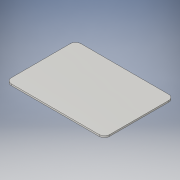
# Autodesk Inventor part: Panel
Saved by Autodesk Inventor 2016 (Build 200138000, 138)
## iProperties
Created: 2016-03-01
Part Number: Panel
Material: Acetal Resin, White
Document SubType Name: Modeling
Designer: agmle
Mass: 839 g
Surface Area: 2036.95 cm^2
Volume: 588.772 cm^3
Density: 1.425 g/cm^3
Appearance: Smooth - White
Author: agmle
Autodesk Inventor part; units mm, degrees
ref_plane "YZ Plane" through (0, 0, 0) normal (1, 0, 0) x (0, 1, 0)
ref_plane "XZ Plane" through (0, 0, 0) normal (0, 1, 0) x (-1, 0, 0)
ref_plane "XY Plane" through (0, 0, 0) normal (0, 0, 1) x (1, 0, 0)
sketch "Sketch1" plane through (0, 0, 0) normal (0, 1, 0) x (-1, 0, 0)
  line L0 (166.5, -132) -> (-166.5, -132)
  line L1 (-186.5, -112) -> (-186.5, 112)
  line L2 (-166.5, 132) -> (166.5, 132)
  line L3 (186.5, 112) -> (186.5, -112)
  line L4 (0, -132) -> (0, 132) construction
  arc A0 (166.5, -132) -> (186.5, -112) centre (166.5, -112) ccw
  arc A1 (-186.5, -112) -> (-166.5, -132) centre (-166.5, -112) ccw
  arc A2 (-166.5, 132) -> (-186.5, 112) centre (-166.5, 112) ccw
  arc A3 (186.5, 112) -> (166.5, 132) centre (166.5, 112) ccw
  point P0 (0, 0)
  point P1 (186.5, -132)
  point P2 (-186.5, -132)
  point P3 (186.5, 132)
  dimension "d0" = 373
  dimension "d1" = 264
  dimension "d2" = 20
  constraints: 10 end point, 8 point on circle, 8 tangent, 6 point on line, 4 centre point, 4 midpoint, 3 equal radius, 2 parallel, 1 horizontal, 1 perpendicular
  measures "d0" distance of point (186.5, -132) point (-186.5, -132)
  measures "d1" distance of point (186.5, 132) point (186.5, -132)
  measures "d2" radius of A0
extrude "Extrusion1" add sketch "Sketch1" along normal blind 6
equation "\"d0\" = Case_Int_Width"
equation "\"d1\" = Case_Int_Height"
equation "\"d3\" = Panel_Thickness"
equation "\"Case_Int_Width\" = 373"
equation "\"Case_Int_Height\" = 264"
equation "\"Panel_Thickness\" = 6"
body "Solid1"
